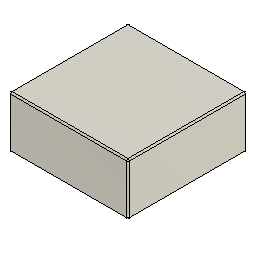
SquareButtonCap-v3 (Autodesk Fusion 360 design; units mm, degrees)
Autodesk Fusion 360 part; units mm, degrees
sketch "Sketch1" plane through (0, 0, 0) normal (0, 0, 1) x (1, 0, 0)
  line L0 (8, -8) -> (-8, -8)
  line L1 (-8, -8) -> (-8, 8)
  line L2 (-8, 8) -> (8, 8)
  line L3 (8, 8) -> (8, -8)
  line L4 (8, -8) -> (-8, 8) construction
  line L5 (-8, -8) -> (8, 8) construction
  line L6 (1.95, -1.95) -> (-1.95, -1.95)
  line L7 (-1.95, -1.95) -> (-1.95, 1.95)
  line L8 (-1.95, 1.95) -> (1.95, 1.95)
  line L9 (1.95, 1.95) -> (1.95, -1.95)
  line L10 (1.95, -1.95) -> (-1.95, 1.95) construction
  line L11 (-1.95, -1.95) -> (1.95, 1.95) construction
  line L12 (5, -5) -> (-5, -5)
  line L13 (-5, -5) -> (-5, 5)
  line L14 (-5, 5) -> (5, 5)
  line L15 (5, 5) -> (5, -5)
  line L16 (5, -5) -> (-5, 5) construction
  line L17 (-5, -5) -> (5, 5) construction
  dimension "d1" = 16
  dimension "d2" = 16
  dimension "d14" = 3.9
  dimension "d15" = 3.9
  dimension "d16" = 10
  dimension "d17" = 10
  constraint horizontal L0
  constraint perpendicular L0 L1
  constraint parallel L0 L2
  constraint parallel L1 L3
  constraint coincident L4 origin
  constraint coincident L5 origin
  constraint horizontal L6
  constraint perpendicular L6 L7
  constraint parallel L6 L8
  constraint parallel L7 L9
  constraint coincident L10 origin
  constraint coincident L11 origin
  constraint horizontal L12
  constraint perpendicular L12 L13
  constraint parallel L12 L14
  constraint parallel L13 L15
  constraint coincident L16 origin
  constraint coincident L17 origin
  measures "d1" distance of L1.end L2.end
  measures "d2" distance of L0.end L1.end
  measures "d14" distance of L7.end L8.end
  measures "d15" distance of L6.end L7.end
  measures "d16" distance of L13.end L14.end
  measures "d17" distance of L12.end L13.end
extrude "Extrude1" add sketch "Sketch1" along normal blind 7 contours L0 L1 L2 L3 | L6 L7 L8 L9 | L12 L13 L14 L15
fillet "Fillet1" radius 0.2 5 faces at (2.6667, -2.6667, 7) (2.6667, -8, 4.6667) (8, 2.6667, 4.6667) (-2.6667, 8, 4.6667) (-8, -2.6667, 4.6667)
extrude "Extrude4" add sketch "Sketch1" against normal blind 1.5 contours L12 L13 L14 L15
extrude "Extrude5" cut 1 faces at (-0.65, 0.65, 0) along direction (0, 0, 1) blind 2
